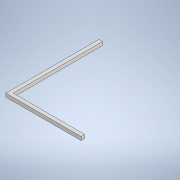
# Autodesk Inventor part: simple corner
Saved by Autodesk Inventor 2020.2 (Build 242310000, 310)
## iProperties
Created: 2021-03-12
Part Number: simple corner
Material: Generic
Document SubType Name: Modeling
Designer: Tarsoly
Density: 1 g/cm^3
Appearance: Default
Author: Tarsoly
Autodesk Inventor part; units mm, degrees
ref_plane "YZ Plane" through (0, 0, 0) normal (1, 0, 0) x (0, 1, 0)
ref_plane "XZ Plane" through (0, 0, 0) normal (0, 1, 0) x (-1, 0, 0)
ref_plane "XY Plane" through (0, 0, 0) normal (0, 0, 1) x (1, 0, 0)
sketch "Sketch1" plane through (0, 0, 0) normal (0, 1, 0) x (-1, 0, 0)
  line L0 (2500, 2500) -> (-2500, 2500)
  line L1 (-2500, 2500) -> (-2500, -2500)
  line L2 (-2500, -2500) -> (2500, -2500)
  line L3 (2500, -2500) -> (2500, 2500)
  line L4 (2500, 2500) -> (-2500, -2500) construction
  line L5 (-2500, 2500) -> (2500, -2500) construction
  line L6 (500, -2500) -> (500, 100)
  line L7 (500, 100) -> (-1600, 100)
  line L8 (-1600, 100) -> (-1600, 0)
  line L9 (-1600, 0) -> (400, 0)
  line L10 (400, 0) -> (400, -2500)
  point P0 (0, 0)
  dimension "d0" = 5000
  dimension "d1" = 5000
  dimension "d7" = 2500
  dimension "d8" = 100
  dimension "d9" = 100
  dimension "d10" = 2000
  dimension "d11" = 2000
  constraints: 22 end point, 5 perpendicular, 2 midpoint, 2 parallel, 2 point on line, 1 horizontal, 1 vertical
  measures "d0" distance of L2.end L1.end
  measures "d1" distance of L1.end L0.end
  measures "d7" distance of L9.end L10.end
  measures "d8" distance of L7.end L8.end
  measures "d9" distance between parallel lines of L10 L6
  measures "d10" distance between parallel lines of L6 L3
  measures "d11" distance of L8.end L9.end
extrude "Extrusion1" add sketch "Sketch1" along normal blind 100 contours L2 L10 L9 L8 L7 L6
body "Solid1"
